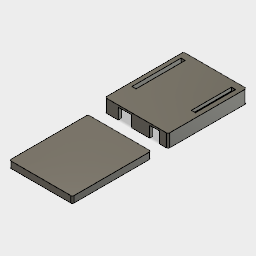
ArduinoCase (Autodesk Fusion 360 design; units mm, degrees)
Autodesk Fusion 360 part; units mm, degrees
sketch "Sketch1" plane through (0, 0, 0) normal (0, 1, 0) x (1, 0, 0)
  line L0 (0, 0) -> (61.1187, 0)
  line L1 (61.1187, 0) -> (61.1187, 76.2)
  line L2 (61.1187, 76.2) -> (0, 76.2)
  line L3 (0, 76.2) -> (0, 0)
  dimension "d1" = 61.1187
  dimension "d2" = 76.2
  constraint horizontal L0
  constraint vertical L1
  constraint horizontal L2
  constraint vertical L3
  constraint coincident L0.start L3.end
  measures "d2" distance of L0.start
extrude "Extrude1" add sketch "Sketch1" against normal blind 6.35 makes body 1
sketch "Sketch2" plane through (0, 0, 0) normal (0, 1, 0) x (-1, 0, 0)
  line L0 (0, -76.2) -> (0, 0)
  line L1 (0, 0) -> (-61.1187, 0)
  line L2 (-61.1187, 0) -> (-61.1187, -76.2)
  line L3 (-61.1187, -76.2) -> (0, -76.2)
  line L4 (-56.515, 0) -> (-41.4337, 0)
  line L5 (-41.4337, 0) -> (-56.515, 0)
  line L6 (-41.4337, 0) -> (-50.0063, 0)
  line L7 (-41.4337, 0) -> (-54.7687, 0)
  line L8 (-54.7687, 0) -> (-54.7687, -14.2875)
  line L9 (-54.7687, -14.2875) -> (-41.4337, -14.2875)
  line L10 (-41.4337, -14.2875) -> (-41.4337, 0)
  dimension "d30" = 19.685
  dimension "d31" = 14.2875
  dimension "d93" = 13.335
  constraint horizontal L6
  constraint horizontal L7
  constraint vertical L8
  constraint horizontal L9
  constraint vertical L10
  measures "d31" distance of L0.end
  measures "d93" distance of L8 L10
extrude "Extrude2" add sketch "Sketch2" along normal blind 12.7 contours L1 L4 L5 L6 L7 L8 L9 L10 bodies 1
sketch "Sketch3" plane through (0, 0, 0) normal (0, 1, 0) x (-1, 0, 0)
  line L0 (-54.7687, 0) -> (-61.1187, 0)
  line L1 (-61.1187, 0) -> (-61.1187, -76.2)
  line L2 (-61.1187, -76.2) -> (0, -76.2)
  line L3 (0, -76.2) -> (0, 0)
  line L4 (0, 0) -> (-41.4337, 0)
  line L5 (0, 0) -> (-27.6225, 0)
  line L6 (-27.6225, 0) -> (-11.1125, 0)
  line L7 (-11.1125, 0) -> (-20.6375, 0)
  line L8 (-11.1125, -12.7) -> (-11.1125, 0)
  line L9 (-54.7687, -14.2875) -> (-54.7687, 0)
  line L10 (-41.4337, 0) -> (-41.4337, -14.2875)
  line L11 (-41.4337, -14.2875) -> (-54.7687, -14.2875)
  line L12 (-11.1125, -12.7) -> (-27.6225, -12.7)
  line L13 (-27.6225, -12.7) -> (-27.6225, 0)
  line L14 (-27.6225, 0) -> (-11.1125, 0)
  line L15 (-11.1125, 0) -> (-11.1125, -12.7)
  dimension "d10" = 27.6225
  dimension "d11" = 16.51
  dimension "d12" = 12.7
  constraint coincident L3.end L4.start
  constraint coincident L5 L3.end
  constraint coincident L4 L3.end
  constraint horizontal L7
  constraint vertical L8
  constraint horizontal L12
  constraint vertical L13
  constraint horizontal L14
  constraint vertical L15
  measures "d12" distance of L3.end
extrude "Extrude3" add sketch "Sketch3" along normal blind 12.7 contours L4 L5 L6 L7 L8 L12 L13 L14 L15 bodies 1
sketch "Sketch12" plane through (0, 0, 0) normal (0, 1, 0) x (-1, 0, 0)
  line L0 (-27.6225, -12.7) -> (-27.6225, 0)
  line L1 (-27.6225, 0) -> (-41.4337, 0)
  line L2 (-41.4337, 0) -> (-41.4337, -14.2875)
  line L3 (-41.4337, -14.2875) -> (-54.7687, -14.2875)
  line L4 (-54.7687, -14.2875) -> (-54.7687, 0)
  line L5 (-54.7687, 0) -> (-61.1187, 0)
  line L6 (-61.1187, 0) -> (-61.1187, -76.2)
  line L7 (-61.1187, -76.2) -> (0, -76.2)
  line L8 (0, -76.2) -> (0, 0)
  line L9 (0, 0) -> (-11.1125, 0)
  line L10 (-11.1125, 0) -> (-11.1125, -12.7)
  line L11 (-11.1125, -12.7) -> (-27.6225, -12.7)
  line L12 (0, 0) -> (-8.7313, 0)
  line L13 (-8.7313, 0) -> (-8.7313, -7.9375)
  line L14 (-8.7313, -7.9375) -> (0, -7.9375)
  line L15 (0, -7.9375) -> (0, 0)
  dimension "d57" = 7.9375
  constraint horizontal L12
  constraint vertical L13
  constraint horizontal L14
  constraint vertical L15
  constraint coincident L8.end L9.start
  measures "d57" distance of L8.end
extrude "Extrude10" add sketch "Sketch12" along normal blind 11.9062 bodies 1
sketch "Sketch13" plane through (0, 11.9062, 0) normal (0, 1, 0) x (-1, 0, 0)
  line L0 (0, 0) -> (-11.1125, 0)
  line L1 (-41.4337, 0) -> (-41.4337, -14.2875)
  line L2 (-41.4337, -14.2875) -> (-54.7687, -14.2875)
  line L3 (-54.7687, -14.2875) -> (-54.7687, 0)
  line L4 (-54.7687, 0) -> (-61.1187, 0)
  line L5 (-61.1187, 0) -> (-61.1187, -76.2)
  line L6 (-61.1187, -76.2) -> (0, -76.2)
  line L7 (0, -76.2) -> (0, 0)
  line L8 (0, -76.2) -> (-7.9375, -76.2)
  line L9 (-7.9375, -76.2) -> (-7.9375, -22.225)
  line L10 (-7.9375, -22.225) -> (0, -22.225)
  line L11 (0, -22.225) -> (0, -76.2)
  line L12 (-61.1187, -76.2) -> (-52.7844, -76.2)
  line L13 (-52.7844, -76.2) -> (-52.7844, -30.9562)
  line L14 (-52.7844, -30.9562) -> (-61.1187, -30.9563)
  line L15 (-61.1187, -30.9563) -> (-61.1187, -76.2)
  line L16 (0, -76.2) -> (-3.9688, -76.2)
  line L17 (-3.9688, -76.2) -> (-3.9688, -22.225)
  line L18 (-3.9688, -22.225) -> (0, -22.225)
  line L19 (0, -22.225) -> (0, -76.2)
  line L20 (0, -76.2) -> (-7.9375, -76.2)
  line L21 (-7.9375, -76.2) -> (-7.9375, -69.85)
  line L22 (-7.9375, -69.85) -> (0, -69.85)
  line L23 (0, -69.85) -> (0, -76.2)
  line L24 (-61.1187, -76.2) -> (-56.7531, -76.2)
  line L25 (-56.7531, -76.2) -> (-56.7531, -30.9563)
  line L26 (-56.7531, -30.9563) -> (-61.1187, -30.9563)
  line L27 (-61.1187, -30.9563) -> (-61.1187, -76.2)
  line L28 (-61.1187, -76.2) -> (-52.7844, -76.2)
  line L29 (-52.7844, -76.2) -> (-52.7844, -69.85)
  line L30 (-52.7844, -69.85) -> (-61.1187, -69.85)
  line L31 (-61.1187, -69.85) -> (-61.1187, -76.2)
  line L32 (-11.1125, 0) -> (-11.1125, -12.7)
  line L33 (-11.1125, -12.7) -> (-27.6225, -12.7)
  line L34 (-27.6225, -12.7) -> (-27.6225, 0)
  line L35 (-27.6225, 0) -> (-41.4337, 0)
  dimension "d60" = 53.975
  dimension "d61" = 7.9375
  dimension "d62" = 45.2437
  dimension "d63" = 8.3344
  dimension "d94" = 53.975
  dimension "d95" = 3.9688
  dimension "d96" = 6.35
  dimension "d97" = 45.2437
  dimension "d98" = 4.3656
  dimension "d99" = 6.35
  constraint horizontal L8
  constraint vertical L9
  constraint horizontal L10
  constraint vertical L11
  constraint horizontal L12
  constraint vertical L13
  constraint horizontal L14
  constraint vertical L15
  constraint horizontal L16
  constraint vertical L17
  constraint horizontal L18
  constraint vertical L19
  constraint horizontal L20
  constraint vertical L21
  constraint horizontal L22
  constraint vertical L23
  constraint horizontal L24
  constraint vertical L25
  constraint horizontal L26
  constraint vertical L27
  constraint coincident L9
  constraint horizontal L28
  constraint vertical L29
  constraint horizontal L30
  constraint vertical L31
  constraint coincident L13
  measures "d62" distance of L0.start
  measures "d97" distance of L0.start
extrude "Extrude11" cut sketch "Sketch13" against normal blind 11.9062 contours L9 L10 L17 L22 | L13 L14 L25 L30 bodies 1
sketch "Sketch14" plane through (0, 0, 0) normal (0, 0, 1) x (1, 0, 0)
  line L0 (0, 11.9062) -> (0, -6.35)
  line L1 (0, -6.35) -> (61.1187, -6.35)
  line L2 (61.1187, -6.35) -> (61.1187, 11.9063)
  line L3 (61.1187, 11.9062) -> (54.7687, 11.9062)
  line L4 (54.7687, 11.9062) -> (54.7687, 12.7)
  line L5 (54.7687, 12.7) -> (41.4337, 12.7)
  line L6 (41.4337, 12.7) -> (41.4337, 11.9062)
  line L7 (27.6225, 12.7) -> (11.1125, 12.7)
  line L8 (11.1125, 12.7) -> (13.0175, 12.7)
  line L9 (13.0175, 12.7) -> (13.0175, 10.795)
  line L10 (13.0175, 10.795) -> (11.1125, 10.795)
  line L11 (11.1125, 10.795) -> (11.1125, 12.7)
  line L12 (27.6225, 12.7) -> (11.1125, 12.7)
  line L13 (11.1125, 12.7) -> (11.1125, 0)
  line L14 (11.1125, 0) -> (27.6225, 0)
  line L15 (27.6225, 0) -> (27.6225, 12.7)
  line L16 (27.6225, 0) -> (25.7175, 0)
  line L17 (25.7175, 0) -> (25.7175, 1.5875)
  line L18 (25.7175, 1.5875) -> (27.6225, 1.5875)
  line L19 (27.6225, 1.5875) -> (27.6225, 0)
  line L20 (13.0175, 10.795) -> (25.7175, 10.795)
  line L21 (25.7175, 10.795) -> (25.7175, 0)
  line L22 (25.7175, 0) -> (13.0175, 0)
  line L23 (13.0175, 0) -> (13.0175, 10.795)
  line L24 (11.1125, 11.9062) -> (0, 11.9062)
  line L25 (41.4337, 11.9062) -> (27.6225, 11.9062)
  line L26 (27.6225, 11.9062) -> (27.6225, 12.7)
  line L27 (11.1125, 12.7) -> (11.1125, 11.9062)
  dimension "d66" = 1.905
  dimension "d67" = 1.905
  dimension "d110" = 12.7
  dimension "d117" = 1.905
  constraint horizontal L8
  constraint vertical L9
  constraint horizontal L10
  constraint vertical L11
  constraint perpendicular L12 L13
  constraint parallel L12 L14
  constraint parallel L13 L15
  constraint perpendicular L11 L12
  constraint horizontal L16
  constraint vertical L17
  constraint horizontal L18
  constraint vertical L19
  constraint horizontal L20
  constraint vertical L21
  constraint horizontal L22
  constraint vertical L23
  measures "d66" distance of origin
  measures "d110" distance of origin
  measures "d117" distance of origin
extrude "Extrude12" cut sketch "Sketch14" against normal blind 9.525 contours L14 L17 L20 L21 L22 L23 bodies 1
sketch "Sketch15" plane through (0, 0, 0) normal (0, 0, 1) x (1, 0, 0)
  line L0 (25.7175, 10.795) -> (25.7175, 0)
  line L1 (25.7175, 0) -> (13.0175, 0)
  line L2 (13.0175, 0) -> (13.0175, 10.795)
  line L3 (13.0175, 10.795) -> (25.7175, 10.795)
  line L4 (0, 11.9062) -> (0, -6.35)
  line L5 (0, -6.35) -> (61.1187, -6.35)
  line L6 (61.1187, -6.35) -> (61.1187, 11.9063)
  line L7 (61.1187, 11.9062) -> (54.7687, 11.9062)
  line L8 (54.7687, 11.9062) -> (54.7687, 12.7)
  line L9 (54.7687, 12.7) -> (41.4337, 12.7)
  line L10 (41.4337, 12.7) -> (41.4337, 11.9062)
  line L11 (27.6225, 12.7) -> (11.1125, 12.7)
  line L12 (41.4337, 12.7) -> (43.3387, 12.7)
  line L13 (43.3387, 12.7) -> (43.3387, 10.795)
  line L14 (43.3387, 10.795) -> (41.4337, 10.795)
  line L15 (41.4337, 10.795) -> (41.4337, 12.7)
  line L16 (54.7687, 12.7) -> (52.8637, 12.7)
  line L17 (52.8637, 12.7) -> (52.8637, 9.525)
  line L18 (52.8637, 9.525) -> (54.7687, 9.525)
  line L19 (54.7687, 9.525) -> (54.7687, 12.7)
  line L20 (43.3387, 12.7) -> (58.7375, 12.7)
  line L21 (11.1125, 11.9062) -> (0, 11.9062)
  line L22 (43.3387, 10.795) -> (52.8637, 10.795)
  line L23 (52.8637, 10.795) -> (52.8637, 0)
  line L24 (52.8637, 0) -> (43.3387, 0)
  line L25 (43.3387, 0) -> (43.3387, 10.795)
  line L26 (56.7531, 0) -> (52.7844, 0)
  line L27 (41.4337, 11.9062) -> (27.6225, 11.9062)
  line L28 (27.6225, 11.9062) -> (27.6225, 12.7)
  line L29 (11.1125, 12.7) -> (11.1125, 11.9062)
  dimension "d72" = 1.905
  dimension "d73" = 1.905
  dimension "d74" = 1.905
  dimension "d75" = 3.175
  constraint horizontal L12
  constraint vertical L13
  constraint horizontal L14
  constraint vertical L15
  constraint horizontal L16
  constraint vertical L17
  constraint horizontal L18
  constraint vertical L19
  constraint horizontal L20
  constraint horizontal L22
  constraint vertical L23
  constraint horizontal L24
  constraint vertical L25
  constraint coincident L17 origin
  constraint coincident origin L26
  measures "d73" distance of origin
extrude "Extrude13" cut sketch "Sketch15" against normal blind 12.7 contours L17 L22 L23 L24 L25 L26 bodies 1
split "Split1" by plane through (0, 0, 0) normal (0, 1, 0) bodies 1 makes body 2 at (22.8865, 11.9062, -41.0104)
move_body "MoveBody1" bodies 1 to x (1, 0, 0) y (0, 1, 0) z (0, 0, 1) at (0, 0, 81.28)
sketch "Sketch16" plane through (0, 0, 0) normal (0, 1, 0) x (-1, 0, 0)
  line L0 (0, 81.28) -> (-61.1187, 81.28)
  line L1 (-61.1187, 81.28) -> (-61.1187, 5.08)
  line L2 (-61.1187, 5.08) -> (0, 5.08)
  line L3 (0, 5.08) -> (0, 81.28)
  line L4 (0, 5.08) -> (-3.175, 5.08)
  line L5 (-3.175, 5.08) -> (-3.175, 8.255)
  line L6 (-3.175, 8.255) -> (0, 8.255)
  line L7 (0, 8.255) -> (0, 5.08)
  line L8 (-61.1187, 81.28) -> (-57.9437, 81.28)
  line L9 (-57.9437, 81.28) -> (-57.9437, 78.105)
  line L10 (-57.9437, 78.105) -> (-61.1187, 78.105)
  line L11 (-61.1187, 78.105) -> (-61.1187, 81.28)
  line L12 (-57.9437, 78.105) -> (-3.175, 78.105)
  line L13 (-3.175, 78.105) -> (-3.175, 8.255)
  line L14 (-3.175, 8.255) -> (-57.9437, 8.255)
  line L15 (-57.9437, 8.255) -> (-57.9437, 78.105)
  dimension "d78" = 3.175
  dimension "d79" = 3.175
  dimension "d80" = 3.175
  dimension "d81" = 3.175
  constraint horizontal L4
  constraint vertical L5
  constraint horizontal L6
  constraint vertical L7
  constraint horizontal L8
  constraint vertical L9
  constraint horizontal L10
  constraint vertical L11
  constraint horizontal L12
  constraint vertical L13
  constraint horizontal L14
  constraint vertical L15
  measures "d79" distance of origin
  measures "d80" distance of origin
extrude "Extrude14" cut sketch "Sketch16" against normal blind 3.175 contours L12 L13 L14 L15 bodies 1
form "Form1" [no effect]
fillet "Fillet1" radius 1.5875 4 edges at (61.1187, -3.175, 81.28) (61.1187, -3.175, 5.08) (0, -3.175, 81.28) (0, -3.175, 5.08) on bodies 1
sketch "Sketch17" plane through (0, 0, 0) normal (0, -1, 0) x (1, 0, 0)
  line L0 (0, 0) -> (0, -76.2)
  line L1 (0, -76.2) -> (61.1187, -76.2)
  line L2 (61.1187, -76.2) -> (61.1187, 0)
  line L3 (13.0175, 0) -> (0, 0)
  line L4 (56.7531, -30.9563) -> (56.7531, -69.85)
  line L5 (56.7531, -69.85) -> (52.7844, -69.85)
  line L6 (52.7844, -69.85) -> (52.7844, -30.9563)
  line L7 (52.7844, -30.9562) -> (56.7531, -30.9563)
  line L8 (7.9375, -69.85) -> (3.9688, -69.85)
  line L9 (3.9688, -69.85) -> (3.9688, -22.225)
  line L10 (3.9688, -22.225) -> (7.9375, -22.225)
  line L11 (7.9375, -22.225) -> (7.9375, -69.85)
  line L12 (13.0175, -9.525) -> (13.0175, 0)
  line L13 (52.8637, -12.7) -> (43.3387, -12.7)
  line L14 (25.7175, 0) -> (25.7175, -9.525)
  line L15 (25.7175, -9.525) -> (13.0175, -9.525)
  line L16 (52.8637, -12.7) -> (52.8637, -15.875)
  line L17 (61.1187, -15.875) -> (25.7175, -15.875)
  line L18 (25.7175, -9.525) -> (25.7175, -12.7)
  line L19 (25.7175, -15.875) -> (25.7175, -12.7)
  line L20 (25.7175, -12.7) -> (0, -12.7)
  line L21 (61.1187, -76.2) -> (61.117, -73.025)
  line L22 (61.117, -73.025) -> (0, -73.025)
  line L23 (52.7844, -69.85) -> (52.7844, -73.025)
  line L24 (7.9375, -69.85) -> (7.9375, -73.025)
  line L25 (56.7531, -69.85) -> (56.7531, -73.025)
  line L26 (3.9688, -69.85) -> (3.9688, -73.025)
  line L27 (56.7531, -30.9563) -> (56.7531, -15.875)
  line L28 (3.9688, -22.225) -> (3.9687, -12.7)
  line L29 (61.1187, 0) -> (52.8637, 0)
  line L30 (52.8637, 0) -> (52.8637, -12.7)
  line L31 (43.3387, -12.7) -> (43.3387, 0)
  line L32 (43.3387, 0) -> (43.3387, -3.175)
  line L33 (25.7175, 0) -> (25.7175, -3.175)
  line L34 (43.3387, -3.175) -> (25.7175, -3.175)
  line L35 (56.7531, -15.875) -> (56.7531, -3.175)
  line L36 (56.7531, -3.175) -> (52.8637, -3.175)
  line L37 (3.9687, -12.7) -> (3.9687, -3.175)
  line L38 (3.9687, -3.175) -> (13.0175, -3.175)
  line L39 (13.0175, -9.525) -> (13.0175, 0)
  dimension "d100" = 3.175
  dimension "d102" = 35.7188
  dimension "d104" = 3.175
  dimension "d105" = 3.175
  dimension "d111" = 3.175
  dimension "d112" = 3.175
  constraint coincident L2
  constraint horizontal L17
  constraint coincident L17
  constraint coincident L0 L3.end
  constraint perpendicular L2 L22
  constraint coincident L22 L0.start
  constraint perpendicular L22 L23
  constraint perpendicular L22 L24
  constraint perpendicular L22 L25
  constraint perpendicular L22 L26
  constraint coincident L0.start L3.end
  constraint perpendicular L17 L27
  constraint coincident L20
  constraint perpendicular L20 L28
  constraint parallel L19 L28
  constraint perpendicular L14 L34
  constraint perpendicular L17 L35
  constraint coincident L30
  constraint perpendicular L30 L36
  constraint perpendicular L20 L37
  constraint coincident L39
  constraint perpendicular L38 L39
  constraint collinear L34 L38
  constraint collinear L34 L36
  measures "d104" distance of L0.start
  measures "d105" distance of L0.start
  measures "d111" distance of L0.start
  measures "d112" distance of L0.start
extrude "Extrude15" cut sketch "Sketch17" against normal blind 9.525 contours L12 L15 L18 L20 L37 L38 L39 | L6 L7 L10 L11 L17 L19 L20 L22 L23 L24 L27 L28 | L8 L22 L24 L26 | L13 L14 L16 L17 L18 L19 L31 L34 | L5 L22 L23 L25 | L16 L17 L30 L35 L36 bodies 2
fillet "Fillet2" radius 1.5875 4 edges at (61.1187, 5.9531, 0) (61.1187, 5.9531, -76.2) (0, 5.9531, -76.2) (0, 5.9531, 0) on bodies 2
move_body "MoveBody2" bodies 1 to x (1, 0, 0) y (0, -1, 0) z (0, 0, -1) at (0, 0, 97.6591)
extrude "Extrude16" add 1 faces at (22.8865, 11.9062, -41.0104) along direction (0, 1, 0) blind 0.7937 on bodies 2 bodies 2
equation "d1 = 2 in + 0.125 in + 0.25 in + ( 1 / 32 ) * 1 in"
equation "d2 = 2 in + ( 3 / 4 ) * 1 in + 0.25 in"
equation "d3 = ( -1 / 4 ) * 1 in"
equation "d8 = ( 7 / 16 ) * 1 in + ( 1 / 16 ) * 1 in"
equation "d10 = ( 3 / 4 ) * 1 in + ( 1 / 8 ) * 1 in + ( 1 / 16 ) * 1 in + 0.15 in"
equation "d11 = ( 1 / 2 ) * 1 in + ( 0.075 * 2 ) * 1 in"
equation "d12 = ( ( 12 / 32 ) * 1 in ) + ( 1 / 8 ) * 1 in"
equation "d13 = ( 1 / 2 ) * 1 in"
equation "d30 = ( ( 3 / 8 ) * 1 in ) + ( 1 / 4 ) * 1 in + ( 0.075 * 2 ) * 1 in"
equation "d31 = ( 1 / 2 ) * 1 in + ( 1 / 16 ) * 1 in"
equation "d57 = ( 5 / 16 ) * 1 in"
equation "d58 = ( 15 / 32 ) * 1 in"
equation "d61 = ( 1 / 4 ) * 1 in + ( 1 / 16 ) * 1 in"
equation "d62 = ( 21 / 32 ) * 1 in + 1 in + 0.125 in"
equation "d63 = ( 3 / 16 ) * 1 in + ( 1 / 8 ) * 1 in + ( 1 / 64 ) * 1 in"
equation "d64 = ( -15 / 32 ) * 1 in"
equation "d66 = ( 1 / 8 ) * 1 in - 0.05 in"
equation "d67 = ( 1 / 8 ) * 1 in - 0.05 in"
equation "d70 = ( -12 / 32 ) * 1 in"
equation "d72 = ( 1 / 8 ) * 1 in - 0.05 in"
equation "d73 = ( 1 / 8 ) * 1 in - 0.05 in"
equation "d74 = ( 1 / 8 ) * 1 in - 0.05 in"
equation "d75 = ( 1 / 8 ) * 1 in"
equation "d76 = ( -16 / 32 ) * 1 in"
equation "d78 = ( 1 / 8 ) * 1 in"
equation "d79 = ( 1 / 8 ) * 1 in"
equation "d80 = ( 1 / 8 ) * 1 in"
equation "d81 = ( 1 / 8 ) * 1 in"
equation "d82 = ( -1 / 8 ) * 1 in"
equation "d84 = ( 1 / 16 ) * 1 in"
equation "d93 = ( 3 / 8 ) * 1 in + ( 0.075 * 2 ) * 1 in"
equation "d94 = 2 in + ( 1 / 8 ) * 1 in"
equation "d95 = ( 1 / 8 ) * 1 in + ( 1 / 32 ) * 1 in"
equation "d96 = ( 1 / 4 ) * 1 in"
equation "d97 = ( 21 / 32 ) * 1 in + 1 in + 0.125 in"
equation "d98 = 0.125 in + ( 1 / 32 ) * 1 in + ( 1 / 64 ) * 1 in"
equation "d99 = ( 1 / 4 ) * 1 in"
equation "d100 = ( 1 / 8 ) * 1 in"
equation "d104 = ( 1 / 8 ) * 1 in"
equation "d105 = ( 1 / 8 ) * 1 in"
equation "d106 = ( -3 / 8 ) * 1 in"
equation "d108 = ( 1 / 16 ) * 1 in"
equation "d110 = ( 1 / 2 ) * 1 in"
equation "d111 = ( 1 / 8 ) * 1 in"
equation "d112 = ( 1 / 8 ) * 1 in"
equation "d115 = ( 1 / 32 ) * 1 in"
